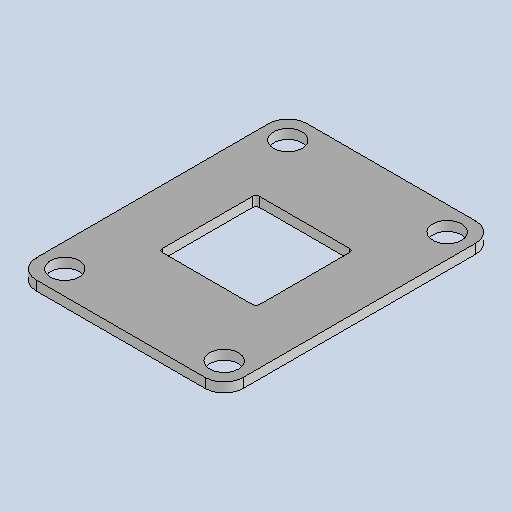
# Autodesk Inventor part: PNS 1669 FDS 1000 FLANGE 3
Saved by Autodesk Inventor 2025.1 (Build 291241020, 241B)
## iProperties
Created: 2025-06-24
Part Number: PNS 1669 FDS 1000 FLANGE 3
Material: Stainless Steel
Document SubType Name: Sheet Metal
Designer: admin
Mass: 103.446 g
Surface Area: 101.897 cm^2
Volume: 12.9307 cm^3
Density: 8 g/cm^3
Flat Pattern Width: 6.5 cm
Flat Pattern Length: 8.5 cm
Flat Pattern Area: 55.25 cm^2
Sheet Metal Rule: AISI304 2mm Die16
Sheet Metal Width: 65.000 mm
Sheet Metal Length: 85.000 mm
Sheet Metal Area: 5525.000 mm^2
Appearance: Default
Author: user
Autodesk Inventor part; units mm, degrees
ref_plane "YZ Plane" through (0, 0, 0) normal (1, 0, 0) x (0, 1, 0)
ref_plane "XZ Plane" through (0, 0, 0) normal (0, 1, 0) x (-1, 0, 0)
ref_plane "XY Plane" through (0, 0, 0) normal (0, 0, 1) x (1, 0, 0)
sketch "Sketch1" plane through (0, 0, 0) normal (0, 0, 1) x (1, 0, 0)
  line L0 (-32.5, -42.5) -> (32.5, -42.5)
  line L1 (32.5, -42.5) -> (32.5, 42.5)
  line L2 (32.5, 42.5) -> (-32.5, 42.5)
  line L3 (-32.5, 42.5) -> (-32.5, -42.5)
  line L4 (-32.5, -42.5) -> (32.5, 42.5) construction
  line L5 (32.5, -42.5) -> (-32.5, 42.5) construction
  line L6 (15.25, -15.25) -> (-15.25, -15.25)
  line L7 (-15.25, -15.25) -> (-15.25, 15.25)
  line L8 (-15.25, 15.25) -> (15.25, 15.25)
  line L9 (15.25, 15.25) -> (15.25, -15.25)
  line L10 (15.25, -15.25) -> (-15.25, 15.25) construction
  line L11 (-15.25, -15.25) -> (15.25, 15.25) construction
  point P0 (0, 0)
  dimension "d154" = 65
  dimension "d155" = 85
  dimension "d172" = 30.5
  measures "d154" distance of L1.end L2.end
  measures "d155" distance of L0.end L1.end
  measures "d172" distance of L7.end L8.end
extrude "Plate5" add sketch "Sketch1" along normal blind 3
sketch "Sketch9" plane through (0, 0, 3) normal (0, 0, 1) x (1, 0, 0)
  circle A0 centre (25, -35) radius 4.5
  line L0 (25, 35) -> (-25, 35) construction
  line L1 (-25, 35) -> (-25, -35) construction
  line L2 (-25, -35) -> (25, -35) construction
  line L3 (25, -35) -> (25, 35) construction
  line L4 (25, 35) -> (-25, -35) construction
  line L5 (-25, 35) -> (25, -35) construction
  circle A1 centre (-25, -35) radius 4.5
  circle A2 centre (25, 35) radius 4.5
  circle A3 centre (-25, 35) radius 4.5
  point P0 (0, 0)
  dimension "d173" = 70
  dimension "d174" = 9
  dimension "d175" = 50
  constraints: 12 end point, 7 coincident, 4 centre point, 3 equal radius, 2 midpoint, 2 parallel, 1 horizontal, 1 perpendicular
  measures "d173" distance of L2.end L0.start
  measures "d174" diameter of A0
  measures "d175" distance of L1.end L2.end
extrude "Cut2" cut sketch "Sketch9" against normal blind 3
fillet "Corner Round1" radius 6 4 edges at (32.5, 42.5, 1.5) (-32.5, 42.5, 1.5) (-32.5, -42.5, 1.5) (32.5, -42.5, 1.5)
fillet "Corner Round2" radius 1 4 edges at (-15.25, 15.25, 1.5) (-15.25, -15.25, 1.5) (15.25, -15.25, 1.5) (15.25, 15.25, 1.5)
body "Solid3"
